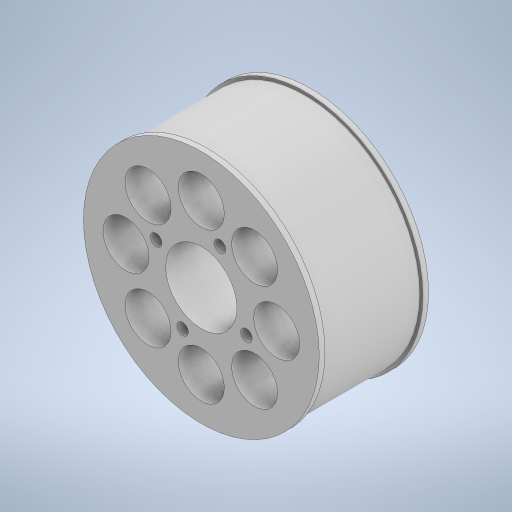
# Autodesk Inventor part: RimV1
Saved by Autodesk Inventor 2024.4 (Build 284460000, 460)
## iProperties
Created: 2026-08-11
Part Number: RimV1
Material: Generic
Document SubType Name: Modeling
Designer: Administrator
Density: 1 g/cm^3
Appearance: Default
Author: Administrator
Autodesk Inventor part; units mm, degrees
ref_plane "YZ Plane" through (0, 0, 0) normal (1, 0, 0) x (0, 1, 0)
ref_plane "XZ Plane" through (0, 0, 0) normal (0, 1, 0) x (-1, 0, 0)
ref_plane "XY Plane" through (0, 0, 0) normal (0, 0, 1) x (1, 0, 0)
sketch "Sketch1" plane through (0, 0, 0) normal (0, 0, 1) x (1, 0, 0)
  circle A0 centre (20.4823, 12.853) radius 3.1
  circle A1 centre (20.4823, 12.853) radius 10
  circle A2 centre (27.0323, 12.853) radius 2
  circle A3 centre (25.1139, 17.4846) radius 2
  circle A4 centre (20.4823, 19.403) radius 2
  circle A5 centre (15.8508, 17.4846) radius 2
  circle A6 centre (13.9323, 12.853) radius 2
  circle A7 centre (15.8508, 8.2215) radius 2
  circle A8 centre (20.4823, 6.303) radius 2
  circle A9 centre (25.1139, 8.2215) radius 2
  line L0 (15.8508, 17.4846) -> (13.9323, 12.853)
  line L1 (14.8916, 15.1688) -> (17.6183, 14.0393)
  line L2 (20.4823, 19.403) -> (25.1139, 17.4846)
  line L3 (22.7981, 18.4438) -> (21.6686, 15.717)
  line L4 (27.0323, 12.853) -> (25.1139, 8.2215)
  line L5 (26.0731, 10.5372) -> (23.3464, 11.6667)
  line L6 (15.8508, 8.2215) -> (20.4823, 6.303)
  line L7 (18.1666, 7.2622) -> (19.296, 9.989)
  circle A10 centre (20.4823, 12.853) radius 4.25
  circle A11 centre (16.5558, 14.4794) radius 0.5
  circle A12 centre (22.1087, 16.7795) radius 0.5
  circle A13 centre (24.4088, 11.2266) radius 0.5
  circle A14 centre (18.8559, 8.9265) radius 0.5
  point P0 (0, 0)
  dimension "d0" = 8.5
  dimension "d1" = 1
  dimension "d2" = 1
  dimension "d3" = 1
  dimension "d4" = 1
  constraints: 16 end point, 15 centre point, 8 point on circle, 4 midpoint, 4 point on line, 1 coincident, 1 perpendicular
  measures "d0" diameter of A10
  measures "d1" diameter of A11
  measures "d2" diameter of A12
  measures "d3" diameter of A13
  measures "d4" diameter of A14
extrude "Extrusion1" add sketch "Sketch1" along normal blind 8.5 contours A0 L3 A12 A10 A13 L5 | A0 L1 A11 A10 A12 L3 | L5 A13 A10 A14 L7 A0 | A0 L7 A14 A10 A11 L1 | A1
sketch "Sketch2" plane through (20.4823, 12.853, 0) normal (0, 0, -1) x (-1, 0, 0)
  circle A0 centre (0, 0) radius 10.25
  circle A1 centre (1.6264, -3.9265) radius 0.5 projected
  circle A2 centre (1.6264, -3.9265) radius 0.5
  circle A3 centre (3.9265, 1.6264) radius 0.5 projected
  circle A4 centre (3.9265, 1.6264) radius 0.5
  circle A5 centre (-1.6264, 3.9265) radius 0.5 projected
  circle A6 centre (-1.6264, 3.9265) radius 0.5
  circle A7 centre (-3.9265, -1.6264) radius 0.5 projected
  circle A8 centre (-3.9265, -1.6264) radius 0.5
  circle A9 centre (6.55, 0) radius 2 projected
  circle A10 centre (6.55, 0) radius 2
  circle A11 centre (4.6315, -4.6315) radius 2 projected
  circle A12 centre (4.6315, -4.6315) radius 2
  circle A13 centre (0, -6.55) radius 2 projected
  circle A14 centre (0, -6.55) radius 2
  circle A15 centre (-4.6315, -4.6315) radius 2 projected
  circle A16 centre (-4.6315, -4.6315) radius 2
  circle A17 centre (-6.55, 0) radius 2 projected
  circle A18 centre (-6.55, 0) radius 2
  circle A19 centre (-4.6315, 4.6315) radius 2 projected
  circle A20 centre (-4.6315, 4.6315) radius 2
  circle A21 centre (0, 6.55) radius 2 projected
  circle A22 centre (0, 6.55) radius 2
  circle A23 centre (4.6315, 4.6315) radius 2 projected
  circle A24 centre (4.6315, 4.6315) radius 2
  circle A25 centre (0, 0) radius 3.1
  point P0 (20.4823, -12.853)
  dimension "d7" = 20.5
  constraints: 14 centre point, 13 coincident
  measures "d7" diameter of A0
extrude "Extrusion2" add sketch "Sketch2" along normal blind 0.5
sketch "Sketch3" plane through (20.4823, 12.853, 8.5) normal (0, 0, 1) x (1, 0, 0)
  circle A0 centre (0, 0) radius 10.25
  circle A1 centre (4.6315, 4.6315) radius 2 projected
  circle A2 centre (4.6315, 4.6315) radius 2
  circle A3 centre (6.55, 0) radius 2 projected
  circle A4 centre (6.55, 0) radius 2
  circle A5 centre (4.6315, -4.6315) radius 2 projected
  circle A6 centre (4.6315, -4.6315) radius 2
  circle A7 centre (0, -6.55) radius 2 projected
  circle A8 centre (0, -6.55) radius 2
  circle A9 centre (-4.6315, -4.6315) radius 2 projected
  circle A10 centre (-4.6315, -4.6315) radius 2
  circle A11 centre (-1.6264, -3.9265) radius 0.5 projected
  circle A12 centre (-1.6264, -3.9265) radius 0.5
  circle A13 centre (-6.55, 0) radius 2 projected
  circle A14 centre (-6.55, 0) radius 2
  circle A15 centre (-3.9265, 1.6264) radius 0.5 projected
  circle A16 centre (-3.9265, 1.6264) radius 0.5
  circle A17 centre (-4.6315, 4.6315) radius 2 projected
  circle A18 centre (-4.6315, 4.6315) radius 2
  circle A19 centre (0, 6.55) radius 2 projected
  circle A20 centre (0, 6.55) radius 2
  circle A21 centre (1.6264, 3.9265) radius 0.5 projected
  circle A22 centre (1.6264, 3.9265) radius 0.5
  circle A23 centre (3.9265, -1.6264) radius 0.5 projected
  circle A24 centre (3.9265, -1.6264) radius 0.5
  circle A25 centre (0, 0) radius 3.1
  point P0 (-20.4823, -12.853)
  dimension "d10" = 20.5
  constraints: 14 centre point, 13 coincident
  measures "d10" diameter of A0
extrude "Extrusion3" add sketch "Sketch3" along normal blind 0.5
body "Solid1"
